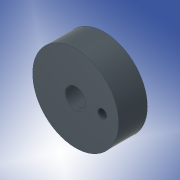
# Autodesk Inventor part: GA002
Saved by Autodesk Inventor 2017 (Build 210142000, 142)
## iProperties
Created: 2017-06-20
Part Number: GA002
Material: ABS Plastic
Document SubType Name: Modeling
Designer: zallen
Density: 1.06 g/cm^3
Appearance: CR Dark Blue
Author: zallen
Autodesk Inventor part; units mm, degrees
ref_plane "YZ Plane" through (0, 0, 0) normal (1, 0, 0) x (0, 1, 0)
ref_plane "XZ Plane" through (0, 0, 0) normal (0, 1, 0) x (-1, 0, 0)
ref_plane "XY Plane" through (0, 0, 0) normal (0, 0, 1) x (1, 0, 0)
sketch "Sketch1" plane through (0, 0, 0) normal (0, 0, 1) x (1, 0, 0)
  circle A0 centre (0, 0) radius 15
  circle A1 centre (0, 0) radius 3.6
  dimension "d0" = 30
  dimension "d1" = 7.2
  constraints: 2 centre point, 2 coincident
  measures "d0" diameter of A0
  measures "d1" diameter of A1
extrude "Extrusion1" add sketch "Sketch1" along normal blind 10
sketch "Sketch2" plane through (0, 0, 10) normal (0, 0, 1) x (1, 0, 0)
  circle A0 centre (9.3, 0) radius 1.5
  circle A1 centre (0, 0) radius 15 construction
  circle A2 centre (0, 0) radius 3.6 construction
  line L0 (3.6, 0) -> (15, 0) construction
  circle A3 centre (0, 0) radius 3.6 construction
  circle A4 centre (0, 0) radius 15 construction
  dimension "d4" = 3
  constraints: 5 horizontal alignment, 2 coincident, 2 end point, 1 centre point, 1 horizontal, 1 midpoint, 4 other
  measures "d4" diameter of A0
extrude "Extrusion2" cut sketch "Sketch2" against normal through all
body "Solid1"
